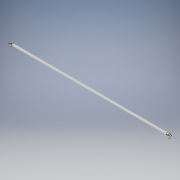
# Autodesk Inventor part: stableBar
Saved by Autodesk Inventor 2018 (Build 220112000, 112)
## iProperties
Created: 2018-03-20
Part Number: stableBar
Material: Generic
Document SubType Name: Sheet Metal
Designer: rochee19
Density: 1 g/cm^3
Sheet Metal Rule: Default
Appearance: Default
Author: rochee19
Autodesk Inventor part; units mm, degrees
ref_plane "YZ Plane" through (0, 0, 0) normal (1, 0, 0) x (0, 1, 0)
ref_plane "XZ Plane" through (0, 0, 0) normal (0, 1, 0) x (-1, 0, 0)
ref_plane "XY Plane" through (0, 0, 0) normal (0, 0, 1) x (1, 0, 0)
sketch "Sketch1" plane through (0, 0, 0) normal (0, 1, 0) x (-1, 0, 0)
  point P0 (0, 0)
sketch "Sketch2" plane through (0, 0, 0) normal (1, 0, 0) x (0, 1, 0)
  circle A0 centre (0, 0) radius 8.3312
  dimension "d0" = 16.6624
  constraints: 1 centre point, 1 coincident
  measures "d0" diameter of A0
sketch "Sketch3" plane through (0, 0, 0) normal (0, 1, 0) x (-1, 0, 0)
  line L0 (0, 0) -> (-38.1, 0)
  line L1 (-38.1, 0) -> (-38.1, -5.08)
  line L2 (-38.1, -5.08) -> (-38.1, 5.08)
  line L3 (0, 0) -> (0, -8.3312)
  line L4 (0, -8.3312) -> (0, 8.3312)
  line L5 (0, 8.3312) -> (-38.1, 5.08)
  line L6 (-38.1, -5.08) -> (0, -8.3312)
  line L7 (-38.1, 0) -> (-22.86, 0)
  line L8 (-38.1, 0) -> (-13.97, 0)
  line L9 (-13.97, 0) -> (-19.05, 0)
  line L10 (-22.1041, -6.445) -> (-22.1041, 6.445)
  line L11 (0, 0) -> (-9.144, 0)
  circle A0 centre (-9.144, 0) radius 6.35
  dimension "d1" = 38.1
  dimension "d2" = 5.08
  dimension "d3" = 10.16
  dimension "d4" = 8.3312
  dimension "d5" = 16.6624
  dimension "d6" = 15.24
  dimension "d7" = 24.13
  dimension "d9" = 9.144
  dimension "d10" = 12.7
  constraints: 24 end point, 8 point on line, 3 vertical, 1 centre point, 1 coincident, 1 horizontal
  measures "d1" distance of L0.start L0.end
  measures "d2" distance of L0.end L1.end
  measures "d3" distance of L1.end L2.end
  measures "d4" distance of L0.start L3.end
  measures "d5" distance of L3.end L4.end
  measures "d6" distance of L0.end L7.end
  measures "d7" distance of L0.end L8.end
  measures "d9" distance of L0.start L11.end
  measures "d10" diameter of A0
extrude "Extrusion1" add sketch "Sketch3" along normal mid plane 1.27 contours L3 L6 L10 L0 A0 | L0 A0 L10 L5 L4
sketch "Sketch4" plane through (0, -0.635, 0) normal (0, -1, 0) x (1, 0, 0)
  circle A0 centre (9.144, 0) radius 6.35 projected
  line L0 (15.494, 0) -> (2.794, 0)
  circle A1 centre (9.144, 0) radius 6.35
  point P0 (0, 0)
  constraints: 2 end point, 2 point on circle, 1 coincident, 1 horizontal, 1 horizontal alignment, 2 other
extrude "Extrusion2" add sketch "Sketch4" along normal mid plane 38.1
sketch "Sketch5" plane through (9.144, 18.415, 0) normal (0, 1, 0) x (1, 0, 0)
  circle A0 centre (0, 0) radius 6.35
  point P0 (-9.144, 0)
  constraints: 1 centre point
extrude "Extrusion3" cut sketch "Sketch5" against normal blind 13.97
sketch "Sketch6" plane through (9.144, 4.445, 0) normal (0, 1, 0) x (1, 0, 0)
  point P0 (-9.144, 0)
sketch "Sketch7" plane through (9.144, 4.445, 0) normal (0, 1, 0) x (1, 0, 0)
  line L0 (0, 0) -> (-1289.6596, 0)
  circle A0 centre (-1289.6596, 0) radius 6.35
  point P0 (-9.144, 0)
  dimension "d17" = 1289.6596
  dimension "d20" = 12.7
  constraints: 2 end point, 1 centre point, 1 coincident, 1 horizontal
  measures "d17" distance of L0.start L0.end
  measures "d20" diameter of A0
extrude "Extrusion4" add sketch "Sketch7" against normal blind 3.81
extrude "Extrusion5" add sketch "Sketch2" against normal blind 1271.27
sketch "Sketch10" plane through (-1280.5156, 0.635, 0) normal (0, -1, 0) x (1, 0, 0)
  circle A0 centre (0, 0) radius 6.35 projected
  line L0 (-6.35, 0) -> (-12.954, 0)
  line L1 (-12.954, 0) -> (-12.954, -6.477)
  line L2 (-12.954, 0) -> (-12.954, 6.477)
  line L3 (9.2456, 8.3312) -> (9.2456, -8.3312) projected
  line L4 (-12.954, -6.477) -> (9.2456, -8.3312)
  line L5 (9.2456, -8.3312) -> (9.2456, 8.3312)
  line L6 (9.2456, 8.3312) -> (-12.954, 6.477)
  point P0 (1280.5156, 0)
  dimension "d37" = 6.604
  dimension "d38" = 6.477
  dimension "d39" = 6.477
  constraints: 12 end point, 2 vertical, 1 collinear, 1 horizontal, 1 horizontal alignment, 1 other
  measures "d37" distance of L0.start L0.end
  measures "d38" distance of L0.end L1.end
  measures "d39" distance of L0.end L2.end
extrude "Extrusion6" add sketch "Sketch10" along normal blind 1.27
sketch "Sketch11" plane through (-1280.5156, 0.635, 0) normal (0, -1, 0) x (1, 0, 0)
  circle A0 centre (0, 0) radius 6.35
  point P0 (1280.5156, 0)
  constraints: 1 centre point
extrude "Extrusion7" add sketch "Sketch11" along normal blind 20.32
fillet "Fillet1" radius 7.62 6 edges at (-1271.27, 6.1114, -5.6621) (-1271.27, 6.1114, 5.6621) (-1271.27, -8.3312, 0) (0, 6.1114, 5.6621) (0, 6.1114, -5.6621) (0, -8.3312, 0)
equation "\"BendRadius\" = Thickness"
equation "\"BendReliefWidth\" = Thickness"
equation "\"BendReliefDepth\" = 0.5 * Thickness"
equation "\"CornerReliefSize\" = 4 * Thickness"
equation "\"MinimumRemnant\" = 2 * Thickness"
equation "\"TransitionRadius\" = BendRadius"
equation "\"JacobiRadiusSize\" = BendRadius"
equation "\"GapSize\" = Thickness"
equation "\"Thickness\" = 3.048"
body "Solid1"
